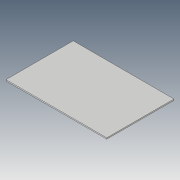
# Autodesk Inventor part: Placchetta
Saved by Autodesk Inventor 2019 (Build 230136000, 136)
## iProperties
Created: 2019-08-01
Part Number: Placchetta
Material: Generic
Document SubType Name: Modeling
Designer: giacomo
Density: 1 g/cm^3
Appearance: Default
Author: giacomo
Autodesk Inventor part; units mm, degrees
ref_plane "YZ Plane" through (0, 0, 0) normal (1, 0, 0) x (0, 1, 0)
ref_plane "XZ Plane" through (0, 0, 0) normal (0, 1, 0) x (-1, 0, 0)
ref_plane "XY Plane" through (0, 0, 0) normal (0, 0, 1) x (1, 0, 0)
sketch "Sketch1" plane through (0, 0, 0) normal (0, 1, 0) x (-1, 0, 0)
  line L0 (5.8371, 10.5387) -> (-27.1629, 10.5387)
  line L1 (-27.1629, 10.5387) -> (-27.1629, -11.4613)
  line L2 (-27.1629, -11.4613) -> (5.8371, -11.4613)
  line L3 (5.8371, -11.4613) -> (5.8371, 10.5387)
  point P0 (0, 0)
  dimension "d0" = 22
  dimension "d1" = 33
  constraints: 8 end point, 2 parallel, 1 horizontal, 1 perpendicular
  measures "d0" distance of L2.end L0.start
  measures "d1" distance of L1.end L2.end
extrude "Extrusion1" add sketch "Sketch1" along normal blind 0.4
body "Solid1"
